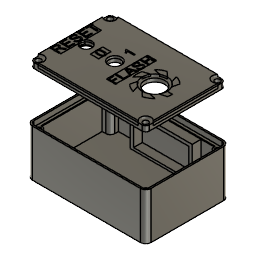
Doomsday box case (Autodesk Fusion 360 design; units mm, degrees)
Autodesk Fusion 360 part; units mm, degrees
note: some values were not read from the file. Chosen so that the rebuilt part matches the saved one: which bodies a step acts on; which face or edge a step refers to.
sketch "Box footprint" plane through (0, 0, 0) normal (0, 0, 1) x (1, 0, 0)
  line L0 (0, 0) -> (130, 0)
  line L1 (130, 0) -> (130, 90)
  line L2 (130, 90) -> (0, 90)
  line L3 (0, 90) -> (0, 0)
  circle A0 centre (125.5, 85.5) radius 1.9
  line L4 (130, 90) -> (121, 90)
  line L5 (121, 90) -> (121, 81)
  line L6 (121, 81) -> (130, 81)
  line L7 (130, 81) -> (130, 90)
  line L8 (0, 81) -> (9, 81)
  line L9 (0, 90) -> (0, 81)
  line L10 (9, 81) -> (9, 90)
  line L11 (9, 90) -> (0, 90)
  circle A1 centre (4.5, 85.5) radius 1.9
  line L12 (121, 0) -> (130, 0)
  line L13 (121, 9) -> (121, 0)
  line L14 (130, 0) -> (130, 9)
  line L15 (130, 9) -> (121, 9)
  circle A2 centre (125.5, 4.5) radius 1.9
  line L16 (0, 0) -> (9, 0)
  line L17 (0, 9) -> (0, 0)
  line L18 (9, 0) -> (9, 9)
  line L19 (9, 9) -> (0, 9)
  circle A3 centre (4.5, 4.5) radius 1.9
  line L20 (4, 4) -> (126, 4) construction
  line L21 (126, 4) -> (126, 86) construction
  line L22 (126, 86) -> (4, 86) construction
  line L23 (4, 86) -> (4, 4) construction
  arc A4 (0, 4) -> (4, 0) centre (4, 4) ccw
  arc A5 (4, 90) -> (0, 86) centre (4, 86) ccw
  arc A6 (130, 86) -> (126, 90) centre (126, 86) ccw
  arc A7 (126, 0) -> (130, 4) centre (126, 4) ccw
  point P0 (125.5, 85.5)
  dimension "d1" = 130
  dimension "d2" = 90
  dimension "d13" = 3.8
  dimension "d14" = 9
  dimension "d15" = 9
  dimension "d19" = 3.8
  dimension "d20" = 9
  dimension "d21" = 9
  dimension "d22" = 3.8
  dimension "d23" = 9
  dimension "d24" = 9
  dimension "d28" = 3.8
  dimension "d29" = 9
  dimension "d30" = 9
  dimension "d125" = 4.5
  dimension "d126" = 4.5
  dimension "d127" = 4.5
  dimension "d128" = 4.5
  dimension "d177" = 4
  dimension "d178" = 4
  dimension "d179" = 4
  dimension "d180" = 4
  constraint horizontal L0
  constraint vertical L1
  constraint horizontal L2
  constraint vertical L3
  constraint coincident L0.start L3.end
  constraint horizontal L4
  constraint perpendicular L4 L5
  constraint parallel L4 L6
  constraint parallel L5 L7
  constraint coincident P0 A0.centre
  constraint horizontal L11
  constraint perpendicular L9 L11
  constraint parallel L8 L11
  constraint parallel L9 L10
  constraint horizontal L15
  constraint perpendicular L13 L15
  constraint parallel L12 L15
  constraint parallel L13 L14
  constraint horizontal L19
  constraint perpendicular L17 L19
  constraint parallel L16 L19
  constraint parallel L17 L18
  constraint coincident L2.end L3.start
  constraint coincident L0.end L1.start
  constraint vertical A1.centre A3.centre
  constraint vertical P0 A2.centre
  constraint horizontal P0 A1.centre
  constraint horizontal A2.centre A3.centre
  constraint horizontal L20
  constraint vertical L21
  constraint horizontal L22
  constraint vertical L23
  constraint coincident L17 A4.start
  constraint coincident L20.start L23.end
  constraint horizontal L20.start A4.start
  constraint vertical L20.start A4.end
  constraint coincident L9 A5.end
  constraint coincident L22.end L23.start
  constraint horizontal L22.end A5.end
  constraint vertical L22.end A5.start
  constraint coincident L4 A6.end
  constraint coincident L21.end L22.start
  constraint vertical L21.end A6.end
  constraint horizontal L21.end A6.start
  constraint coincident L12 A7.start
  constraint coincident L20.end L21.start
  constraint vertical L20.end A7.start
  constraint horizontal L20.end A7.end
  measures "d1" distance of L0.start L0.end
  measures "d2" distance of L0.start L2.end
  measures "d13" diameter of A0
  measures "d14" distance of L5.end L6.end
  measures "d15" distance of L4.end L5.end
  measures "d19" diameter of A1
  measures "d20" distance of L8.start L8.end
  measures "d21" distance of L2.end L8.start
  measures "d22" diameter of A2
  measures "d23" distance of L12.start L0.end
  measures "d24" distance of L13.start L12.start
  measures "d28" diameter of A3
  measures "d29" distance of L0.start L16.end
  measures "d30" distance of L17.start L0.start
  measures "d125" distance of A1.centre L9
  measures "d126" distance of L1 P0
  measures "d127" distance of L0 A2.centre
  measures "d128" distance of L2 P0
  measures "d177" distance of L0 L20
  measures "d178" distance of L3 L23
  measures "d179" distance of L1 L21
  measures "d180" distance of L2 L22
extrude "Extrude1" add sketch "Box footprint" against normal blind 4 contours L0 L3 L16 L17 L18 L19 A4 | L0 L1 L2 L3 L5 L6 L8 L10 L13 L15 L18 L19 | L0 L1 L12 L13 L14 L15 A7 | L2 L3 L8 L9 L10 L11 A5 | L1 L2 L4 L5 L6 L7 A6 | A0 | A1 | A2 | A3 makes body 1
extrude "Extrude5" add sketch "Box footprint" along normal blind 2 contours L0 L3 L16 L17 L18 L19 A4 | L0 L1 L12 L13 L14 L15 A7 | L2 L3 L8 L9 L10 L11 A5 | L1 L2 L4 L5 L6 L7 A6 | A0 | A1 | A2 | A3 bodies 1
sketch "Lid outline" plane through (0, 0, -4) normal (0, 0, -1) x (1, 0, 0)
  arc A0 (4, 0) -> (0, -4) centre (4, -4) ccw
  arc A1 (0, -86) -> (4, -90) centre (4, -86) ccw
  arc A2 (126, -90) -> (130, -86) centre (126, -86) ccw
  arc A3 (130, -4) -> (126, 0) centre (126, -4) ccw
  line L0 (126, 0) -> (4, 0)
  line L1 (0, -4) -> (0, -86)
  line L2 (4, -90) -> (126, -90)
  line L3 (130, -86) -> (130, -4)
  line L4 (-0.2, -4) -> (-0.2, -86)
  arc A4 (-0.2, -86) -> (4, -90.2) centre (4, -86) ccw
  line L5 (4, -90.2) -> (126, -90.2)
  arc A5 (126, -90.2) -> (130.2, -86) centre (126, -86) ccw
  line L6 (130.2, -86) -> (130.2, -4)
  arc A6 (130.2, -4) -> (126, 0.2) centre (126, -4) ccw
  line L7 (126, 0.2) -> (4, 0.2)
  arc A7 (4, 0.2) -> (-0.2, -4) centre (4, -4) ccw
  line L8 (126, 2) -> (4, 2)
  arc A8 (4, 2) -> (-2, -4) centre (4, -4) ccw
  line L9 (-2, -4) -> (-2, -86)
  arc A9 (-2, -86) -> (4, -92) centre (4, -86) ccw
  line L10 (4, -92) -> (126, -92)
  arc A10 (126, -92) -> (132, -86) centre (126, -86) ccw
  line L11 (132, -86) -> (132, -4)
  arc A11 (132, -4) -> (126, 2) centre (126, -4) ccw
  line L12 (121, -9) -> (121, 0.2)
  line L13 (121, -9) -> (130.2, -9)
  line L14 (121, -81) -> (121, -90.2)
  line L15 (121, -81) -> (130.2, -81)
  line L16 (9, -81) -> (9, -90.2)
  line L17 (9, -81) -> (-0.2, -81)
  line L18 (9, -9) -> (-0.2, -9)
  line L19 (9, -9) -> (9, 0.2)
  circle A12 centre (4.5, -85.5) radius 1.9
  circle A13 centre (4.5, -4.5) radius 1.9
  circle A14 centre (125.5, -4.5) radius 1.9
  circle A15 centre (125.5, -85.5) radius 1.9
  point P0 (9, -9)
  point P1 (9, -81)
  point P2 (121, -81)
  point P3 (121, -9)
  dimension "d181" = 0.2
  dimension "d182" = 2
  constraint coincident A3.end L0.start
  constraint coincident A0.start L0.end
  constraint coincident A0.end L1.start
  constraint coincident A1.start L1.end
  constraint coincident A1.end L2.start
  constraint coincident A2.start L2.end
  constraint coincident A2.end L3.start
  constraint coincident A3.start L3.end
  constraint coincident P3 L12.start
  constraint coincident L7 L12.end
  constraint perpendicular L7 L12
  constraint coincident L6 L13.end
  constraint perpendicular L6 L13
  constraint coincident P2 L14.start
  constraint coincident L5 L14.end
  constraint perpendicular L5 L14
  constraint coincident L6 L15.end
  constraint perpendicular L6 L15
  constraint coincident P1 L16.start
  constraint coincident L5 L16.end
  constraint perpendicular L5 L16
  constraint coincident L4 L17.end
  constraint perpendicular L4 L17
  constraint coincident P0 L18.start
  constraint coincident L4 L18.end
  constraint perpendicular L4 L18
  constraint coincident L7 L19.end
  constraint perpendicular L7 L19
extrude "Extrude8" add sketch "Lid outline" against normal blind 49 separate body contours L8 A8 L9 A9 L10 A10 L11 A11 makes body 2
sketch "Lid screw holes" plane through (0, 0, 45) normal (0, 0, 1) x (-1, 0, 0)
  circle A0 centre (-4.5, -85.5) radius 1.7
  circle A1 centre (-4.5, -4.5) radius 1.7
  circle A2 centre (-125.5, -4.5) radius 1.7
  circle A3 centre (-125.5, -85.5) radius 1.7
  circle A4 centre (-125.5, -85.5) radius 3
  circle A5 centre (-125.5, -4.5) radius 3
  circle A6 centre (-4.5, -4.5) radius 3
  circle A7 centre (-4.5, -85.5) radius 3
  arc A8 (0.2, -4) -> (-4, 0.2) centre (-4, -4) ccw
  line L0 (0.2, -4) -> (0.2, -86)
  arc A9 (-4, -90.2) -> (0.2, -86) centre (-4, -86) ccw
  line L1 (-4, -90.2) -> (-126, -90.2)
  arc A10 (-130.2, -86) -> (-126, -90.2) centre (-126, -86) ccw
  line L2 (-130.2, -86) -> (-130.2, -4)
  arc A11 (-126, 0.2) -> (-130.2, -4) centre (-126, -4) ccw
  line L3 (-126, 0.2) -> (-4, 0.2)
  arc A12 (-126, 2) -> (-132, -4) centre (-126, -4) ccw
  line L4 (-132, -4) -> (-132, -86)
  arc A13 (-132, -86) -> (-126, -92) centre (-126, -86) ccw
  line L5 (-126, -92) -> (-4, -92)
  arc A14 (-4, -92) -> (2, -86) centre (-4, -86) ccw
  line L6 (2, -86) -> (2, -4)
  arc A15 (2, -4) -> (-4, 2) centre (-4, -4) ccw
  line L7 (-4, 2) -> (-126, 2)
  point P0 (-4.5, -85.5)
  point P1 (-4.5, -4.5)
  point P2 (-125.5, -4.5)
  point P3 (-125.5, -85.5)
  point P4 (-4, -76)
  point P5 (-4, -76)
  dimension "d63" = 3.4
  dimension "d64" = 3.4
  dimension "d65" = 3.4
  dimension "d66" = 3.4
  dimension "d67" = 6
  dimension "d68" = 6
  dimension "d69" = 6
  dimension "d70" = 6
  constraint coincident P1 A1.centre
  constraint concentric A3 A4
  constraint concentric A2 A5
  constraint concentric A1 A6
  constraint concentric A0 A7
  constraint coincident P0 A0.centre
  constraint coincident P2 A2.centre
  constraint coincident P3 A3.centre
  measures "d63" diameter of A0
  measures "d64" diameter of A1
  measures "d65" diameter of A2
  measures "d66" diameter of A3
  measures "d67" diameter of A4
  measures "d68" diameter of A5
  measures "d69" diameter of A6
  measures "d70" diameter of A7
extrude "Extrude9" add sketch "Lid screw holes" along normal blind 4 contours A0 | A1 | A2 | A3 | A4 | A5 | A6 | A7 | A8 L0 A9 L1 A10 L2 A11 L3 | A12 L4 A13 L5 A14 L6 A15 L7 bodies 2
extrude "Extrude16" add sketch "Lid outline" against normal up to surface (43 mm away) from surface at -6 contours A0 L0 L1 L18 L19 | A0 L0 L1 L4 L7 A7 L18 L19 | A3 L0 L3 L6 A6 L7 L12 L13 | A3 L0 L3 L12 L13 | A1 L1 L2 L16 L17 | A1 L1 L2 L4 A4 L5 L16 L17 | A2 L2 L3 L5 A5 L6 L14 L15 | A2 L2 L3 L14 L15 | A12 | A13 | A14 | A15 bodies 2
extrude "Extrude17" cut sketch "Lid outline" against normal blind 12 from surface at -6 contours A12 | A13 | A14 | A15 bodies 2
chamfer "Chamfer3" distance 0.8 angle 45 4 edges at (2.7286, 3.8129, 2) (123.7286, 3.8129, 2) (123.7286, 84.8129, 2) (2.7286, 84.8129, 2) on bodies 2
extrude "Extrude18" cut sketch "Lid screw holes" against normal up to surface (6 mm away) from surface at -43 contours A0 | A1 | A2 | A3 bodies 1
extrude "Extrude19" cut sketch "Lid screw holes" along normal blind 4 from surface at -49 contours A4 | A5 | A6 | A7 bodies 1
extrude "Extrude20" add sketch "Lid screw holes" along normal blind 0.2 from surface at -45 contours A0 | A1 | A2 | A3 bodies 1
sketch "Lid rebate" plane through (0, 0, 45) normal (0, 0, -1) x (1, 0, 0)
  line L0 (121, -2.8) -> (9, -2.8)
  line L1 (9, -87.2) -> (121, -87.2)
  line L2 (2.8, -9) -> (2.8, -81)
  line L3 (127.2, -81) -> (127.2, -9)
  line L4 (9, -81) -> (9, -90.2)
  line L5 (9, -81) -> (-0.2, -81)
  line L6 (4, -90.2) -> (126, -90.2)
  line L7 (-0.2, -4) -> (-0.2, -86)
  line L8 (9, -9) -> (-0.2, -9)
  line L9 (9, -9) -> (9, 0.2)
  line L10 (126, 0.2) -> (4, 0.2)
  line L11 (121, -9) -> (121, 0.2)
  line L12 (121, -9) -> (130.2, -9)
  line L13 (130.2, -86) -> (130.2, -4)
  line L14 (121, -81) -> (121, -90.2)
  line L15 (121, -81) -> (130.2, -81)
  dimension "d189" = 3
  dimension "d190" = 3
  dimension "d191" = 3
  dimension "d192" = 3
  constraint coincident L0.start L11
  constraint coincident L0.end L9
  constraint coincident L2.start L8
  constraint coincident L2.end L5
  constraint coincident L1.start L4
  constraint coincident L1.end L14
  constraint coincident L3.start L15
  constraint coincident L3.end L12
  measures "d189" distance of L1 L6
  measures "d190" distance of L3 L13
  measures "d191" distance of L0 L10
  measures "d192" distance of L2 L7
sketch "Lip" plane through (0, 0, 0) normal (0, 0, 1) x (-1, 0, 0)
  line L0 (0, -9) -> (-9, -9)
  line L1 (-9, -9) -> (-9, 0)
  line L2 (-9, 0) -> (-121, 0)
  line L3 (-121, 0) -> (-121, -9)
  line L4 (-121, -9) -> (-130, -9)
  line L5 (-130, -9) -> (-130, -81)
  line L6 (-130, -81) -> (-121, -81)
  line L7 (-121, -81) -> (-121, -90)
  line L8 (-121, -90) -> (-9, -90)
  line L9 (-9, -90) -> (-9, -81)
  line L10 (-9, -81) -> (0, -81)
  line L11 (0, -81) -> (0, -9)
  line L12 (-121, -2.8) -> (-9, -2.8)
  line L13 (-2.8, -9) -> (-2.8, -81)
  line L14 (-127.2, -81) -> (-127.2, -9)
  line L15 (-9, -87.2) -> (-121, -87.2)
extrude "Extrude22" add sketch "Lip" against normal up to surface (2 mm away) from surface at 2 contours L0 L10 L11 L13 | L1 L2 L3 L12 | L7 L8 L9 L15 | L4 L5 L6 L14 bodies 1
extrude "Extrude23" add sketch "Lid rebate" against normal blind 4 from surface at 43 contours L0 L9 L10 L11 | L3 L12 L13 L15 | L2 L5 L7 L8 | L1 L4 L6 L14 bodies 2
chamfer "Chamfer2" distance 3 angle 45 4 edges at (65, 87.2, 6) (2.8, 45, 6) (127.2, 45, 6) (65, 2.8, 6) on bodies 2
fillet "Fillet3" radius 5 4 edges at (121, 9, 23.5) (9, 9, 23.5) (9, 81, 23.5) (121, 81, 23.5) on bodies 2
fillet "Fillet4" radius 5 12 edges at (5.9, 81, 2) (9, 84.1, 2) (121, 84.1, 2) (124.1, 81, 2) (124.1, 9, 2) (121, 5.9, 2) (9, 5.9, 2) (5.9, 9, 2) (9, 81, 1) (121, 81, 1) (121, 9, 1) (9, 9, 1) on bodies 1
move_body "Align2" bodies 2 to x (1, 0, 0) y (0, -1, 0) z (0, 0, -1) at (0, 90, 49)
sketch "Sketch10" plane through (0, 0, 2) normal (0, 0, 1) x (-1, 0, 0)
  line L0 (-4, -281) -> (-2.8, -281)
  line L1 (-2.8, -281) -> (-2.8, -209)
  line L2 (-2.8, -209) -> (-4, -209)
  arc A0 (-9, -204) -> (-4, -209) centre (-4, -204) ccw
  line L3 (-9, -204) -> (-9, -202.8)
  line L4 (-9, -202.8) -> (-121, -202.8)
  line L5 (-121, -202.8) -> (-121, -204)
  arc A1 (-126, -209) -> (-121, -204) centre (-126, -204) ccw
  line L6 (-126, -209) -> (-127.2, -209)
  line L7 (-127.2, -209) -> (-127.2, -281)
  line L8 (-127.2, -281) -> (-126, -281)
  arc A2 (-121, -286) -> (-126, -281) centre (-126, -286) ccw
  line L9 (-121, -286) -> (-121, -287.2)
  line L10 (-121, -287.2) -> (-9, -287.2)
  line L11 (-9, -287.2) -> (-9, -286)
  arc A3 (-4, -281) -> (-9, -286) centre (-4, -286) ccw
move_body "Move4" bodies 1 to x (1, 0, 0) y (0, 1, 0) z (0, 0, 1) at (0, 0, 110)
move_body "Move5" bodies 1 to x (1, 0, 0) y (0, -1, 0) z (0, 0, -1) at (0, 90, 220)
sketch "Sketch11" plane through (0, 0, 110) normal (0, 0, -1) x (1, 0, 0)
  line L0 (2.8, -9) -> (2.8, -81)
  line L1 (2.8, -81) -> (4, -81)
  arc A0 (9, -86) -> (4, -81) centre (4, -86) ccw
  line L2 (9, -86) -> (9, -87.2)
  line L3 (9, -87.2) -> (121, -87.2)
  line L4 (121, -87.2) -> (121, -86)
  arc A1 (126, -81) -> (121, -86) centre (126, -86) ccw
  line L5 (126, -81) -> (127.2, -81)
  line L6 (127.2, -81) -> (127.2, -9)
  line L7 (127.2, -9) -> (126, -9)
  arc A2 (121, -4) -> (126, -9) centre (126, -4) ccw
  line L8 (121, -4) -> (121, -2.8)
  line L9 (121, -2.8) -> (9, -2.8)
  line L10 (9, -2.8) -> (9, -4)
  arc A3 (4, -9) -> (9, -4) centre (4, -4) ccw
  line L11 (4, -9) -> (2.8, -9)
  line L12 (2.8, -45) -> (127.2, -45) construction
  circle A4 centre (95.2, -45) radius 11.25
  circle A5 centre (50.2, -45) radius 6.65
  circle A6 centre (17.8, -45) radius 6.5
  dimension "d193" = 22.5
  dimension "d194" = 32
  dimension "d195" = 13.3
  dimension "d196" = 45
  dimension "d197" = 13
  dimension "d199" = 15
  constraint midpoint L0 L12.start
  constraint midpoint L6 L12.end
  constraint coincident L12 A4.centre
  constraint coincident L12 A5.centre
  constraint coincident L12 A6.centre
  measures "d193" diameter of A4
  measures "d194" distance of L6 A4.centre
  measures "d195" diameter of A5
  measures "d196" distance of A4.centre A5.centre
  measures "d197" diameter of A6
  measures "d199" distance of L0 A6.centre
extrude "Extrude26" cut sketch "Sketch11" against normal through all contours A4 | A5 | A6 bodies 1
sketch "Text layer" plane through (0, 0, 114) normal (0, 0, 1) x (1, 0, 0)
  line L0 (4, 0) -> (126, 0)
  line L1 (130, 4) -> (130, 86)
  line L2 (126, 90) -> (4, 90)
  line L3 (0, 86) -> (0, 4)
  circle A0 centre (4.5, 4.5) radius 3
  circle A1 centre (125.5, 4.5) radius 3
  circle A2 centre (125.5, 85.5) radius 3
  circle A3 centre (4.5, 85.5) radius 3
  circle A4 centre (17.8, 45) radius 6.5
  circle A5 centre (50.2, 45) radius 6.65
  circle A6 centre (95.2, 45) radius 11.25
  arc A7 (130, 86) -> (126, 90) centre (126, 86) ccw
  arc A8 (4, 90) -> (0, 86) centre (4, 86) ccw
  arc A9 (0, 4) -> (4, 0) centre (4, 4) ccw
  arc A10 (126, 0) -> (130, 4) centre (126, 4) ccw
sketch "Sketch12" plane through (0, 90.2, 0) normal (0, -1, 0) x (1, 0, 0)
  line L0 (121, 43) -> (9, 43)
  line L1 (9, 43) -> (9, 4)
  line L2 (9, 4) -> (121, 4)
  line L3 (121, 4) -> (121, 43)
  line L4 (65, 4) -> (65, 43) construction
  line L5 (32.2407, 43) -> (102.2407, 43)
  line L6 (102.2407, 43) -> (102.2407, 3)
  line L7 (102.2407, 3) -> (32.2407, 3)
  line L8 (32.2407, 3) -> (32.2407, 43)
  line L9 (98.4606, 39.22) -> (98.4606, 6.78)
  line L10 (98.4606, 6.78) -> (36.0207, 6.78)
  line L11 (36.0207, 6.78) -> (36.0207, 39.22)
  line L12 (36.0207, 39.22) -> (98.4606, 39.22)
  dimension "d201" = 40
  dimension "d202" = 70
  dimension "d203" = 3.78
  constraint midpoint L2 L4.start
  constraint midpoint L0 L4.end
  constraint horizontal L5
  constraint vertical L6
  constraint horizontal L7
  constraint vertical L8
  constraint coincident L0 L5.start
  measures "d201" distance of L5.end L6.end
  measures "d202" distance of L5.start L5.end
extrude "Extrude27" add sketch "Sketch12" along normal blind 10 contours L0 L2 L5 L6 L8 bodies 2
ref_plane "WorkPlane1" through (65, 45, 116) normal (0, 0, 1) x (-1, 0, 0)
sketch "Sketch13" plane through (0, 0, 116) normal (0, 0, 1) x (1, 0, 0)
  circle A0 centre (17.8, 45) radius 6.5
  circle A1 centre (50.2, 45) radius 6.65
  circle A2 centre (95.2, 45) radius 11.25
  circle A3 centre (4.5, 4.5) radius 3
  circle A4 centre (125.5, 4.5) radius 3
  circle A5 centre (125.5, 85.5) radius 3
  circle A6 centre (4.5, 85.5) radius 3
  arc A7 (130, 86) -> (126, 90) centre (126, 86) ccw
  line L0 (126, 90) -> (4, 90)
  arc A8 (4, 90) -> (0, 86) centre (4, 86) ccw
  line L1 (0, 86) -> (0, 4)
  arc A9 (0, 4) -> (4, 0) centre (4, 4) ccw
  line L2 (4, 0) -> (126, 0)
  arc A10 (126, 0) -> (130, 4) centre (126, 4) ccw
  line L3 (130, 4) -> (130, 86)
  circle A11 centre (4.5, 85.5) radius 6
  circle A12 centre (125.5, 85.5) radius 6
  circle A13 centre (125.5, 4.5) radius 6
  circle A14 centre (4.5, 4.5) radius 6
  circle A15 centre (95.2, 45) radius 14
  circle A16 centre (50.2, 45) radius 7.5
  circle A17 centre (17.8, 45) radius 6.5
  line L4 (50.2, 45) -> (34.2, 45) construction
  line L5 (38.8108, 51.9483) -> (29.5892, 51.9483)
  line L6 (29.5892, 51.9483) -> (29.5892, 38.0517) construction
  line L7 (29.5892, 38.0517) -> (38.8108, 38.0517) construction
  line L8 (38.8108, 38.0517) -> (38.8108, 51.9483) construction
  line L9 (38.8108, 51.9483) -> (29.5892, 38.0517) construction
  line L10 (29.5892, 51.9483) -> (38.8108, 38.0517) construction
  line L11 (50.2, 45) -> (50.2, 61) construction
  line L12 (38.8108, 38.0517) -> (38.8108, 51.9483) construction
  line L13 (38.8108, 51.9483) -> (29.5892, 51.9483) construction
  line L14 (29.5892, 51.9483) -> (29.5892, 38.0517) construction
  line L15 (29.5892, 38.0517) -> (38.8108, 38.0517) construction
  line L16 (55, 67.9858) -> (45.4, 67.9858)
  line L17 (45.4, 67.9858) -> (45.4, 54.0142)
  line L18 (45.4, 54.0142) -> (55, 54.0142)
  line L19 (55, 54.0142) -> (55, 67.9858)
  line L20 (55, 67.9858) -> (45.4, 54.0142) construction
  line L21 (45.4, 67.9858) -> (55, 54.0142) construction
  line L22 (55, 54.0142) -> (55, 67.9858) construction
  line L23 (55, 67.9858) -> (45.4, 67.9858) construction
  line L24 (45.4, 67.9858) -> (45.4, 54.0142) construction
  line L25 (45.4, 54.0142) -> (55, 54.0142) construction
  circle A18 centre (95.2, 45) radius 20
  line L26 (17.8, 45) -> (7.8, 45) construction
  line L27 (95.2, 45) -> (120.2, 45)
  line L28 (81.2047, 45.3634) -> (75.9153, 39.6989)
  line L29 (82.898, 38.3171) -> (81.1496, 30.7668)
  line L30 (87.8877, 33.0614) -> (90.1486, 25.6484)
  line L31 (94.8366, 31.0047) -> (100.5011, 25.7153)
  line L32 (101.8829, 32.698) -> (109.4332, 30.9496)
  line L33 (107.1386, 37.6877) -> (114.5516, 39.9486)
  line L34 (109.1953, 44.6366) -> (114.4847, 50.3011)
  line L35 (107.502, 51.6829) -> (109.2504, 59.2332)
  line L36 (102.5123, 56.9386) -> (100.2514, 64.3516)
  line L37 (95.5634, 58.9953) -> (89.8989, 64.2847)
  line L38 (88.5171, 57.302) -> (80.9668, 59.0504)
  line L39 (83.2614, 52.3123) -> (75.8484, 50.0514)
  line L40 (95.2, 45) -> (68.2025, 45.3687) construction
  line L41 (71.1991, 76.5066) -> (65.206, 76.5066) construction
  line L42 (65.206, 76.5066) -> (65.206, 14.2308) construction
  line L43 (65.206, 14.2308) -> (71.1991, 14.2308) construction
  line L44 (71.1991, 14.2308) -> (71.1991, 76.5066) construction
  line L45 (71.1991, 76.5066) -> (65.206, 14.2308) construction
  line L46 (65.206, 76.5066) -> (71.1991, 14.2308) construction
  line L47 (71.1991, 14.2308) -> (71.1991, 76.5066) construction
  line L48 (71.1991, 76.5066) -> (65.206, 76.5066) construction
  line L49 (65.206, 76.5066) -> (65.206, 14.2308) construction
  line L50 (65.206, 14.2308) -> (71.1991, 14.2308) construction
  line L51 (15.8, 53.7033) -> (-0.2, 53.7033) construction
  line L52 (-0.2, 53.7033) -> (-0.2, 36.2967) construction
  line L53 (-0.2, 36.2967) -> (15.8, 36.2967) construction
  line L54 (15.8, 36.2967) -> (15.8, 53.7033) construction
  line L55 (15.8, 53.7033) -> (-0.2, 36.2967) construction
  line L56 (-0.2, 53.7033) -> (15.8, 36.2967) construction
  line L57 (7.8, 36.2967) -> (7.8, 53.7033) construction
  line L58 (7.8, 53.7033) -> (3.8472, 53.7033) construction
  line L59 (3.8472, 53.7033) -> (3.8472, 36.2967) construction
  line L60 (3.8472, 36.2967) -> (7.8, 36.2967) construction
  line L61 (62.8128, 22.9818) -> (73.0514, 22.9818)
  line L62 (29.5892, 38.0517) -> (38.8108, 38.0517)
  line L63 (38.8108, 38.0517) -> (38.8108, 51.9483)
  line L64 (38.8108, 51.9483) -> (29.5892, 51.9483)
  line L65 (29.5892, 51.9483) -> (29.5892, 38.0517)
  line L66 (63, 69) -> (73.0514, 69)
  line L67 (73.0514, 69) -> (73.0514, 22.9818)
  line L68 (73.0514, 22.9818) -> (63, 22.9818)
  line L69 (63, 22.9818) -> (63, 69)
  line L70 (0, 67.369) -> (12.5481, 67.369)
  line L71 (12.5481, 67.369) -> (12.5481, 21.7783)
  line L72 (12.5481, 21.7783) -> (0, 21.7783)
  line L73 (0, 21.7783) -> (0, 67.369)
  point P0 (4.5, 85.5)
  point P1 (4.5, 4.5)
  point P2 (125.5, 4.5)
  point P3 (125.5, 85.5)
  point P4 (34.2, 45)
  point P5 (50.2, 61)
  point P6 (7.8, 45)
  point P7 (120.2, 45)
  point P8 (68.2025, 45.3687)
  point P9 (7.8, 45)
  dimension "d207" = 12
  dimension "d208" = 12
  dimension "d209" = 12
  dimension "d210" = 12
  dimension "d211" = 28
  dimension "d212" = 15
  dimension "d217" = 10
  dimension "d219" = 10
  dimension "d221" = 6
  dimension "d222" = 16
  dimension "d223" = 16
  dimension "d224" = 10
  dimension "d225" = 25
  dimension "d227" = 360
  dimension "d228" = 27
  dimension "d229" = 10
  dimension "d231" = 10
  text T0 "0" font "Arial" height 10 align centre middle in box 13.8965 x 9.2216 at (38.8108, 38.0517) x (0, 1) y (-1, 0) spacing 1.1
  text T1 "1" font "Arial" height 10 align centre middle in box 13.9716 x 9.6 at (55, 54.0142) x (0, 1) y (-1, 0) spacing 1.1
  text T2 "FLASH" font "Arial" height 10 align centre middle in box 62.2759 x 5.9931 at (71.1991, 14.2308) x (0, 1) y (-1, 0) spacing 1.1
  text T3 "RESET" font "Arial" height 10 align centre middle in box 17.4066 x 3.9528 at (7.8, 36.2967) x (0, 1) y (-1, 0) spacing 1.1
  constraint concentric A6 A11
  constraint concentric A5 A12
  constraint concentric A4 A13
  constraint coincident P1 A3.centre
  constraint concentric A2 A15
  constraint concentric A1 A16
  constraint concentric A0 A17
  constraint coincident A1.centre A16.centre
  constraint horizontal L4
  constraint horizontal L5
  constraint perpendicular L5 L6
  constraint parallel L5 L7
  constraint parallel L6 L8
  constraint coincident L9 P4
  constraint coincident L10 P4
  constraint coincident P4 L4.end
  constraint coincident L5.start
  constraint coincident L6.end
  constraint horizontal L16
  constraint perpendicular L16 L17
  constraint parallel L16 L18
  constraint parallel L17 L19
  constraint coincident L20 P5
  constraint coincident L21 P5
  constraint coincident P5 L11.end
  constraint coincident L16.start
  constraint coincident L17.end
  constraint coincident A0.centre A17.centre
  constraint horizontal L26
  constraint coincident P9 P6
  constraint coincident A2.centre A15.centre
  constraint horizontal L27
  constraint coincident P7 L27.end
  constraint coincident A15 L28.start
  constraint coincident A18 L28.end
  constraint horizontal L41
  constraint perpendicular L41 L42
  constraint parallel L41 L43
  constraint parallel L42 L44
  constraint coincident L45 P8
  constraint coincident L46 P8
  constraint coincident P8 L40.end
  constraint coincident L41.start
  constraint coincident L42.end
  constraint horizontal L51
  constraint perpendicular L51 L52
  constraint parallel L51 L53
  constraint parallel L52 L54
  constraint coincident L55 P9
  constraint coincident L56 P9
  constraint midpoint L51
  constraint coincident L53
  constraint horizontal L61
  constraint horizontal L62
  constraint vertical L63
  constraint horizontal L64
  constraint vertical L65
  constraint horizontal L66
  constraint vertical L67
  constraint horizontal L68
  constraint vertical L69
  constraint horizontal L70
  constraint vertical L71
  constraint horizontal L72
  constraint vertical L73
  constraint coincident L1 L70.start
  measures "d207" diameter of A11
  measures "d208" diameter of A12
  measures "d209" diameter of A13
  measures "d210" diameter of A14
  measures "d211" diameter of A15
  measures "d212" diameter of A16
  measures "d222" distance of A1.centre P4
  measures "d223" distance of A1.centre P5
  measures "d224" distance of A0.centre P9
  measures "d225" distance of A2.centre P7
  measures "d228" distance of A2.centre P8
extrude "Extrude28" add sketch "Sketch13" sketch "Sketch13" against normal blind 4 separate body contours A0 L1 A17 L70 L71 L72 L73 | L5 L62 L63 L64 L65 | L16 L17 L18 L19 | L61 L66 L67 L68 L69 of sketch 2 text T2 makes body 3 at (48.6, 58.6714, 116) makes body 4 at (32.6631, 47.3161, 116) makes body 5 at (3.772, 44.5642, 116) makes body 6 at (66.3505, 46.3007, 116)
extrude "Extrude29" add sketch "Sketch13" against normal blind 5 separate body contours A0 L0 L1 L2 L3 A11 A12 A13 A14 A17 L70 L71 L72 | A0 L1 A17 L70 L71 L72 L73 | A15 A18 L27 L34 L35 | A15 A18 L35 L36 | A15 A18 L27 L33 L34 | A18 L27 L34 | A15 A18 L36 L37 | A15 A18 L32 L33 | A15 A18 L37 L38 | A15 A18 L31 L32 | A15 A18 L38 L39 | A15 A18 L30 L31 | A15 A18 L28 L39 | A15 A18 L29 L30 | A15 A18 L28 L29 | L5 L62 L63 L64 L65 | L16 L17 L18 L19 makes body 7
extrude "Extrude30" add sketch "Sketch13" against normal blind 2 separate body contours A15 A18 L35 L36 | A15 A18 L27 L33 L34 | A15 A18 L37 L38 | A15 A18 L31 L32 | A15 A18 L28 L39 | A15 A18 L29 L30 makes body 8 at (111.2301, 43.7043, 116) makes body 9 at (77.2533, 45.9055, 116) makes body 10 at (103.3892, 29.0049, 116) makes body 11 at (106.8436, 58.6869, 116) makes body 12 at (87.0108, 60.9951, 116) makes body 13 at (83.5564, 31.3131, 116)
extrude "Extrude31" cut sketch "Sketch13" against normal blind 2 text T3 T0 T1 T2 bodies 6 5 4 7
extrude "Extrude32" add sketch "Sketch13" against normal blind 2 separate body text T2 T0 T1 T3 makes body 14 at (5.9623, 32.3211, 116) makes body 15 at (6.0324, 46.1387, 116) makes body 16 at (48.506, 62.8417, 115.3333) makes body 17 at (68.3549, 23.1986, 116) makes body 18 at (68.298, 60.5765, 116) makes body 19 at (68.4113, 54.5115, 116) makes body 20 at (68.5004, 41.3692, 116) makes body 21 at (69.8692, 31.7848, 114.6667) makes body 22 at (35.1442, 42.6081, 116) makes body 23 at (5.9623, 52.1901, 116) makes body 24 at (7.8836, 64.6417, 116) makes body 25 at (6.01, 21.6089, 116)
extrude "Extrude14" [suppressed]
hidden bodies 3
equation "d1 = Length"
equation "d2 = Width"
equation "d13 = ScrewHoleRadius"
equation "d19 = ScrewHoleRadius"
equation "d22 = ScrewHoleRadius"
equation "d28 = ScrewHoleRadius"
equation "d31 = -Coverthickness"
equation "d40 = StudLength"
equation "d63 = ScrewClearHole"
equation "d64 = ScrewClearHole"
equation "d65 = ScrewClearHole"
equation "d66 = ScrewClearHole"
equation "d67 = ScrewHeadRadius"
equation "d68 = ScrewHeadRadius"
equation "d69 = ScrewHeadRadius"
equation "d70 = ScrewHeadRadius"
equation "d71 = Coverthickness"
equation "Width = 90 mm"
equation "Length = 130 mm"
equation "Height = 45 mm"
equation "ScrewHoleRadius = 3.8 mm" comment "2.7 for M3 screws"
equation "ScrewHeadRadius = 6 mm" comment "6mm for cap head M3 hex screws"
equation "clearance = 0.2 mm" comment "between lid and body"
equation "WallThickness = 1.8 mm"
equation "Coverthickness = 4 mm"
equation "d107 = -Coverthickness - Height"
equation "ScrewClearHole = 3.4 mm" comment "3.4 for an m3 screw"
equation "StudLength = 2 mm"
equation "d110 = -Coverthickness - StudLength"
equation "d181 = clearance"
equation "d182 = clearance + WallThickness"
equation "d208 = d207"
equation "d209 = d207"
equation "d210 = d207"
equation "d218 = 0"
equation "d220 = 1"
equation "d230 = 'FLASH'"
equation "d232 = 'RESET'"
named bodies: "Lid", "Main Body"
